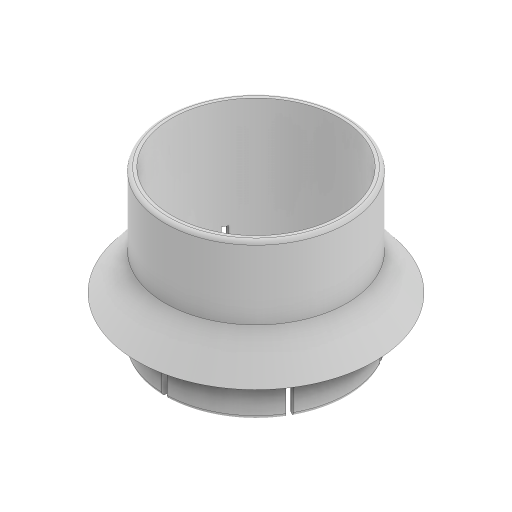
# Autodesk Inventor part: top-ventilation-tube-adapter-100.9mmID-to-95mmID
Saved by Autodesk Inventor 2023 (Build 270158000, 158)
## iProperties
Created: 2024-07-10
Part Number: top-ventilation-tube-adapter-100.9mmID-to-95mmID
Material: Generic
Document SubType Name: Modeling
Designer: N.Vladimirov
Density: 1 g/cm^3
Appearance: Default
Author: N.Vladimirov
Autodesk Inventor part; units mm, degrees
ref_plane "YZ Plane" through (0, 0, 0) normal (1, 0, 0) x (0, 1, 0)
ref_plane "XZ Plane" through (0, 0, 0) normal (0, 1, 0) x (-1, 0, 0)
ref_plane "XY Plane" through (0, 0, 0) normal (0, 0, 1) x (1, 0, 0)
sketch "Sketch1" plane through (0, 0, 0) normal (0, 0, 1) x (1, 0, 0)
  line L0 (-50.35, 0) -> (-46.35, 0)
  line L1 (-46.35, 0) -> (-46.35, -25)
  line L2 (-46.35, -25) -> (-48.35, -25)
  line L3 (-50.35, -23) -> (-50.35, 0)
  line L4 (-46.35, 20) -> (-50, 20)
  line L5 (-50, 20) -> (-50, 58)
  line L6 (-48, 60) -> (-46.35, 60)
  line L7 (-46.35, 60) -> (-46.35, 20)
  line L8 (-50.35, 0) -> (-65.35, 0)
  line L9 (-65.35, 0) -> (-50, 20)
  line L10 (-46.35, 20) -> (-46.35, 0)
  arc A0 (-48, 60) -> (-50, 58) centre (-48, 58) ccw
  arc A1 (-50.35, -23) -> (-48.35, -25) centre (-48.35, -23) ccw
  line L11 (0, -42.5799) -> (0, 77.5799) projected
  point P0 (0, 0)
  point P1 (-50.35, -25)
  point P2 (-50, 60)
  point P3 (-48.35, 0)
  dimension "d4" = 4
  dimension "d5" = 25
  dimension "d7" = 40
  dimension "d8" = 15
  dimension "d9" = 50.35
  dimension "d10" = 2
  dimension "d12" = 20
  dimension "d20" = 50
  constraints: 22 end point, 5 point on line, 4 parallel, 4 point on circle, 4 tangent, 3 horizontal, 2 centre point, 2 perpendicular, 1 equal radius, 1 midpoint, 1 vertical
  measures "d4" distance of L1.end point (-50.35, -25)
  measures "d5" distance of L0.end L1.end
  measures "d7" distance of L4.end point (-50, 60)
  measures "d8" distance of L0.start L8.end
  measures "d9" distance of point (0, 0) L0.start
  measures "d10" radius of A0
  measures "d12" distance from line of point (-48.35, 0) L4
  measures "d20" distance between parallel lines of L11 L5
revolve "Revolution1" add sketch "Sketch1" angle 360 about axis through (0, -10, 0) along (0, 1, 0)
sketch "Sketch2" plane through (0, -25, 0) normal (0, -1, 0) x (1, 0, 0)
  line L0 (1.5, 41.35) -> (-1.5, 41.35)
  line L1 (-1.5, 41.35) -> (-1.5, 51.35)
  line L2 (-1.5, 51.35) -> (1.5, 51.35)
  line L3 (1.5, 51.35) -> (1.5, 41.35)
  circle A0 centre (0, 0) radius 46.35 projected
  line L4 (1.5, 41.35) -> (-1.5, 51.35) construction
  line L5 (-1.5, 41.35) -> (1.5, 51.35) construction
  point P0 (0, 46.35)
  dimension "d13" = 3
  dimension "d14" = 10
  constraints: 12 end point, 2 midpoint, 2 parallel, 1 horizontal, 1 perpendicular, 1 vertical alignment, 1 other
  measures "d13" distance of L1.end L2.end
  measures "d14" distance of L0.end L1.end
extrude "Extrusion1" cut sketch "Sketch2" against normal blind 25 contours L0 L1 A0 L3 | A0 L1 L2 L3 picked at (-0.1667, 43.0158)
pattern_circular "Circular Pattern1" count 6 over 360 about axis through (0, -10, 0) along (0, 1, 0) of "Extrusion1"
body "Solid1"
